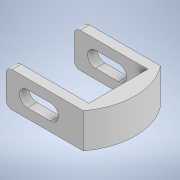
# Autodesk Inventor part: yystop
Saved by Autodesk Inventor 2022 (Build 260153000, 153)
## iProperties
Created: 2022-07-18
Part Number: yystop
Material: Genérico
Document SubType Name: Modeling
Designer: JK
Density: 1 g/cm^3
Appearance: Valor por defecto
Author: JK
Autodesk Inventor part; units mm, degrees
ref_plane "YZ Plane" through (0, 0, 0) normal (1, 0, 0) x (0, 1, 0)
ref_plane "XZ Plane" through (0, 0, 0) normal (0, 1, 0) x (-1, 0, 0)
ref_plane "XY Plane" through (0, 0, 0) normal (0, 0, 1) x (1, 0, 0)
sketch "Boceto1" plane through (0, 0, 0) normal (0, 1, 0) x (-1, 0, 0)
  line L0 (-14.8958, 21.4303) -> (7.8042, 21.4303)
  line L1 (7.8042, 21.4303) -> (7.8042, -5.2697)
  line L2 (7.8042, -5.2697) -> (-14.8958, -5.2697)
  line L3 (-14.8958, -5.2697) -> (-14.8958, 21.4303)
  line L4 (-14.8958, 21.4303) -> (7.8042, -5.2697) construction
  line L5 (7.8042, 21.4303) -> (-14.8958, -5.2697) construction
  arc A0 (-14.8958, 21.4303) -> (-14.8958, -5.2697) centre (2.3487, 8.0803) ccw
  line L6 (7.8042, 15.4612) -> (7.8042, 21.4303)
  line L7 (-13.6958, 18.2303) -> (6.6042, 18.2303)
  line L8 (6.6042, 18.2303) -> (6.6042, -2.0697)
  line L9 (6.6042, -2.0697) -> (-13.6958, -2.0697)
  line L10 (-13.6958, -2.0697) -> (-13.6958, 18.2303)
  line L11 (-13.6958, 18.2303) -> (6.6042, -2.0697) construction
  line L12 (6.6042, 18.2303) -> (-13.6958, -2.0697) construction
  line L13 (7.8042, 21.4303) -> (11.6042, 21.4303)
  line L14 (11.6042, 21.4303) -> (11.6042, -5.2697)
  line L15 (11.6042, -5.2697) -> (7.8042, -5.2697)
  line L16 (7.8042, -5.2697) -> (7.8042, 21.4303)
  line L17 (7.8042, 21.4303) -> (6.6042, 21.4303)
  line L18 (6.6042, 21.4303) -> (6.6042, -5.2697)
  line L19 (6.6042, -5.2697) -> (7.8042, -5.2697)
  line L20 (7.8042, -5.2697) -> (7.8042, 21.4303)
  line L21 (11.6042, -5.2697) -> (6.6042, -5.2697)
  line L22 (6.6042, -5.2697) -> (6.6042, -2.0697)
  line L23 (6.6042, -2.0697) -> (11.6042, -2.0697)
  line L24 (11.6042, -2.0697) -> (11.6042, -5.2697)
  line L25 (11.6042, 21.4303) -> (6.6042, 21.4303)
  line L26 (6.6042, 21.4303) -> (6.6042, 18.2303)
  line L27 (6.6042, 18.2303) -> (11.6042, 18.2303)
  line L28 (11.6042, 18.2303) -> (11.6042, 21.4303)
  point P0 (-3.5458, 8.0803)
  point P1 (6.6042, -2.0697)
  point P2 (6.6042, 18.2303)
  point P3 (6.6042, 18.2303)
  point P4 (6.6042, -2.0697)
  dimension "d4" = 20.3
  dimension "d5" = 3.2
  dimension "d6" = 1.2
  dimension "d7" = 20.3
  dimension "d14" = 5
  constraints: 58 end point, 12 parallel, 6 horizontal, 6 perpendicular, 4 midpoint, 3 point on line, 2 point on circle, 1 centre point
  measures "d4" distance of L7.end L8.end
  measures "d5" distance between parallel lines of L7 L0
  measures "d6" distance between parallel lines of L10 L3
  measures "d7" distance of L7.start L7.end
  measures "d14" distance between parallel lines of L14 L18
extrude "Extrusión1" add sketch "Boceto1" along normal blind 12 contours L0 L18 L7 L10 L9 L2 L3 | L3 A0 | L0 L1 L27 L18 | L13 L14 L27 L1 | L18 L23 L1 L2 | L1 L23 L14 L15
sketch "Boceto2" plane through (-6.6042, 0, 21.4303) normal (0, 0, 1) x (1, 0, 0)
  circle A0 centre (2.3, 6) radius 2.7
  line L0 (-5, 0) -> (21.5, 0) projected
  circle A1 centre (10.3, 6) radius 2.7
  line L1 (2.3, 3.3) -> (10.3, 3.3)
  line L2 (10.3, 3.3) -> (10.3, 8.7)
  line L3 (10.3, 8.7) -> (2.3, 8.7)
  line L4 (2.3, 8.7) -> (2.3, 3.3)
  point P0 (6.6042, 0)
  point P1 (20.3, 0)
  dimension "d10" = 5.4
  dimension "d11" = 6
  dimension "d12" = 10
  dimension "d13" = 8
  constraints: 8 end point, 2 horizontal, 2 parallel, 2 tangent, 1 centre point, 1 perpendicular, 1 vertical alignment, 3 other
  measures "d11" distance from line of L0 point (2.3, 6)
  measures "d12" horizontal distance of point (20.3, 0) A1.centre
  measures "d13" distance of L1.start L1.end
extrude "Extrusión2" cut sketch "Boceto2" against normal through all
fillet "Empalme1" radius 2 4 edges at (-11.6042, 0, 19.8303) (-11.6042, 12, 19.8303) (-11.6042, 0, -3.6697) (-11.6042, 12, -3.6697)
